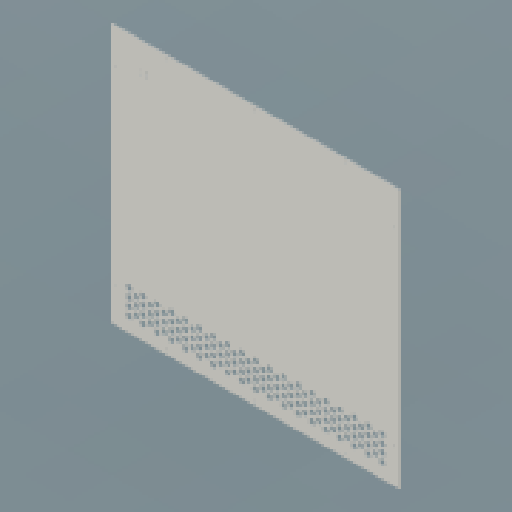
# Autodesk Inventor part: Rear Panel
Saved by Autodesk Inventor 2023.2 (Build 272271000, 271)
## iProperties
Created: 2023-02-06
Part Number: Rear Panel
Material: Aluminum 6061
Document SubType Name: Modeling
Designer: remop
Density: 2.7 g/cm^3
Appearance: Aluminum - Flat
Author: remop
Autodesk Inventor part; units mm, degrees
(part 1 of 2)
ref_plane "YZ Plane" through (0, 0, 0) normal (1, 0, 0) x (0, 1, 0)
ref_plane "XZ Plane" through (0, 0, 0) normal (0, 1, 0) x (-1, 0, 0)
ref_plane "XY Plane" through (0, 0, 0) normal (0, 0, 1) x (1, 0, 0)
sketch "Sketch1" plane through (0, 0, 0) normal (0, 0, 1) x (1, 0, 0)
  line L0 (287.336, -253.0124) -> (287.336, 226.9876) projected
  line L1 (287.336, 226.9876) -> (289.336, 226.9876) projected
  line L2 (289.336, -253.0124) -> (289.336, 226.9876) projected
  line L3 (287.336, -253.0124) -> (289.336, -253.0124) projected
  line L4 (-242.664, 226.9876) -> (-242.664, -253.0124) projected
  line L5 (-242.664, -253.0124) -> (-244.664, -253.0124) projected
  line L6 (-244.664, 226.9876) -> (-244.664, -253.0124) projected
  line L7 (-242.664, 226.9876) -> (-244.664, 226.9876) projected
  line L8 (287.336, 226.9876) -> (-242.664, 226.9876)
  line L9 (-242.664, -253.0124) -> (287.336, -253.0124)
  circle A0 centre (187.336, 219.4876) radius 1.75
  circle A1 centre (-142.664, 219.4876) radius 1.75
  circle A2 centre (22.336, 219.4876) radius 1.75
  circle A3 centre (187.336, -245.5124) radius 1.75
  circle A4 centre (22.336, -245.5124) radius 1.75
  circle A5 centre (-142.664, -245.5124) radius 1.75
  circle A6 centre (279.836, 161.9876) radius 1.75
  circle A7 centre (279.836, -188.0124) radius 1.75
  circle A8 centre (-235.164, -188.0124) radius 1.75
  circle A9 centre (-235.164, 161.9876) radius 1.75
  point P0 (0, 0)
  point P1 (22.336, 226.9876)
  dimension "d0" = 7.5
  dimension "d1" = 100
  dimension "d2" = 100
  dimension "d3" = 3.5
  dimension "d4" = 7.5
  dimension "d7" = 65
  dimension "d8" = 65
  dimension "d10" = 7.5
  dimension "d11" = 7.5
  constraints: 10 centre point, 9 equal radius, 6 horizontal alignment, 6 vertical alignment, 4 end point, 1 horizontal, 1 midpoint, 1 parallel
  measures "d0" distance from line of A0.centre L8
  measures "d1" distance from line of L0 A0.centre
  measures "d2" distance from line of L4 A1.centre
  measures "d3" diameter of A2
  measures "d4" distance from line of L9 A3.centre
  measures "d7" distance from line of A7.centre L9
  measures "d8" distance from line of L8 A6.centre
  measures "d10" distance from line of L4 A9.centre
  measures "d11" distance from line of L0 A6.centre
extrude "Extrusion1" add sketch "Sketch1" against normal blind 2
sketch "Sketch2" plane through (0, 0, 0) normal (0, 0, 1) x (1, 0, 0)
  line L0 (-204.6641, 162.9876) -> (-216.6641, 162.9876) projected
  line L1 (-204.6641, 162.9876) -> (-204.6641, 184.9876) projected
  line L2 (-216.6641, 184.9876) -> (-204.6641, 184.9876) projected
  line L3 (-216.6641, 162.9876) -> (-216.6641, 184.9876) projected
  line L4 (70.3359, 162.9876) -> (-204.6641, 162.9876) projected
  line L5 (70.3359, 162.9876) -> (70.3359, 184.9876) projected
  line L6 (-204.6641, 184.9876) -> (70.3359, 184.9876) projected
  line L7 (-204.6641, 162.9876) -> (-204.6641, 184.9876) projected
  point P0 (0, 0)
  point P1 (-209.6641, 177.4876)
  point P2 (-209.6641, 170.4876)
  point P3 (-199.6641, 170.4876)
  point P4 (-199.6641, 177.4876)
  dimension "d12" = 7
  dimension "d13" = 10
  dimension "d14" = 7.5
  dimension "d15" = 7
  constraints: 2 horizontal alignment, 2 vertical alignment
  measures "d12" distance of point (-199.664, 170.488) point (-199.664, 177.488)
  measures "d13" distance of point (-199.664, 177.488) point (-209.664, 177.488)
  measures "d14" distance from line of L2 point (-209.664, 177.488)
  measures "d15" distance from line of L3 point (-209.664, 177.488)
hole "Hole1" at (-209.6641, 177.4876, 0) at (-209.6641, 170.4876, 0) at (-199.6641, 170.4876, 0) at (-199.6641, 177.4876, 0) direction (0, 0, -1) diameter 3.5 end through all
sketch "Sketch4" plane through (0, 0, -2) normal (0, 0, -1) x (-1, 0, 0)
  circle A0 centre (199.6641, 170.4876) radius 1.75 projected
  circle A1 centre (209.6641, 177.4876) radius 1.75 projected
  circle A2 centre (209.6641, 170.4876) radius 1.75 projected
  circle A3 centre (199.6641, 177.4876) radius 1.75 projected
  line L0 (244.664, 226.9876) -> (-289.336, 226.9876) projected
  line L1 (-289.336, 226.9876) -> (-289.336, -253.0124) projected
  line L2 (-289.336, -253.0124) -> (244.664, -253.0124) projected
  line L3 (244.664, -253.0124) -> (244.664, 226.9876) projected
  circle A4 centre (235.164, 161.9876) radius 1.75 projected
  circle A5 centre (-279.836, -188.0124) radius 1.75 projected
  circle A6 centre (-279.836, 161.9876) radius 1.75 projected
  circle A7 centre (142.664, -245.5124) radius 1.75 projected
  circle A8 centre (-22.336, -245.5124) radius 1.75 projected
  circle A9 centre (-187.336, -245.5124) radius 1.75 projected
  circle A10 centre (-22.336, 219.4876) radius 1.75 projected
  circle A11 centre (142.664, 219.4876) radius 1.75 projected
  circle A12 centre (-187.336, 219.4876) radius 1.75 projected
  circle A13 centre (235.164, -188.0124) radius 1.75 projected
  line L4 (-250.5625, -226.0124) -> (-253.4493, -231.0124)
  line L5 (-253.4493, -231.0124) -> (-259.2228, -231.0124)
  line L6 (-259.2228, -231.0124) -> (-262.1095, -226.0124)
  line L7 (-262.1095, -226.0124) -> (-259.2228, -221.0124)
  line L8 (-259.2228, -221.0124) -> (-253.4493, -221.0124)
  line L9 (-253.4493, -221.0124) -> (-250.5625, -226.0124)
  line L10 (-246.2324, -223.5124) -> (-249.1191, -218.5124)
  line L11 (-249.1191, -218.5124) -> (-246.2324, -213.5124)
  line L12 (-246.2324, -213.5124) -> (-240.4589, -213.5124)
  line L13 (-240.4589, -213.5124) -> (-237.5721, -218.5124)
  line L14 (-237.5721, -218.5124) -> (-240.4589, -223.5124)
  line L15 (-240.4589, -223.5124) -> (-246.2324, -223.5124)
  line L16 (-253.4493, -216.0124) -> (-259.2228, -216.0124)
  line L17 (-259.2228, -216.0124) -> (-262.1095, -211.0124)
  line L18 (-262.1095, -211.0124) -> (-259.2228, -206.0124)
  line L19 (-259.2228, -206.0124) -> (-253.4493, -206.0124)
  line L20 (-253.4493, -206.0124) -> (-250.5625, -211.0124)
  line L21 (-250.5625, -211.0124) -> (-253.4493, -216.0124)
  line L22 (-246.2324, -198.5124) -> (-240.4589, -198.5124)
  line L23 (-249.1191, -203.5124) -> (-246.2324, -198.5124)
  line L24 (-240.4589, -198.5124) -> (-237.5721, -203.5124)
  line L25 (-250.5625, -196.0124) -> (-253.4493, -201.0124)
  line L26 (-253.4493, -191.0124) -> (-250.5625, -196.0124)
  line L27 (-253.4493, -201.0124) -> (-259.2228, -201.0124)
  line L28 (-259.2228, -191.0124) -> (-253.4493, -191.0124)
  line L29 (-262.1095, -196.0124) -> (-259.2228, -191.0124)
  line L30 (-259.2228, -201.0124) -> (-262.1095, -196.0124)
  line L31 (-237.5721, -203.5124) -> (-240.4589, -208.5124)
  line L32 (-240.4589, -208.5124) -> (-246.2324, -208.5124)
  line L33 (-246.2324, -208.5124) -> (-249.1191, -203.5124)
  line L34 (-246.2324, -183.5124) -> (-240.4589, -183.5124)
  line L35 (-249.1191, -188.5124) -> (-246.2324, -183.5124)
  line L36 (-240.4589, -183.5124) -> (-237.5721, -188.5124)
  line L37 (-250.5625, -181.0124) -> (-253.4493, -186.0124)
  line L38 (-253.4493, -176.0124) -> (-250.5625, -181.0124)
  line L39 (-253.4493, -186.0124) -> (-259.2228, -186.0124)
  line L40 (-259.2228, -176.0124) -> (-253.4493, -176.0124)
  line L41 (-262.1095, -181.0124) -> (-259.2228, -176.0124)
  line L42 (-259.2228, -186.0124) -> (-262.1095, -181.0124)
  line L43 (-237.5721, -188.5124) -> (-240.4589, -193.5124)
  line L44 (-240.4589, -193.5124) -> (-246.2324, -193.5124)
  line L45 (-246.2324, -193.5124) -> (-249.1191, -188.5124)
  line L46 (-227.4493, -176.0124) -> (-224.5625, -181.0124)
  line L47 (-233.2228, -176.0124) -> (-227.4493, -176.0124)
  line L48 (-236.1095, -181.0124) -> (-233.2228, -176.0124)
  line L49 (-214.4589, -208.5124) -> (-220.2324, -208.5124)
  line L50 (-220.2324, -198.5124) -> (-214.4589, -198.5124)
  line L51 (-211.5721, -188.5124) -> (-214.4589, -193.5124)
  line L52 (-214.4589, -193.5124) -> (-220.2324, -193.5124)
  line L53 (-214.4589, -183.5124) -> (-211.5721, -188.5124)
  line L54 (-220.2324, -183.5124) -> (-214.4589, -183.5124)
  line L55 (-220.2324, -208.5124) -> (-223.1191, -203.5124)
  line L56 (-223.1191, -203.5124) -> (-220.2324, -198.5124)
  line L57 (-220.2324, -193.5124) -> (-223.1191, -188.5124)
  line L58 (-223.1191, -188.5124) -> (-220.2324, -183.5124)
  line L59 (-224.5625, -211.0124) -> (-227.4493, -216.0124)
  line L60 (-227.4493, -221.0124) -> (-224.5625, -226.0124)
  line L61 (-224.5625, -226.0124) -> (-227.4493, -231.0124)
  line L62 (-233.2228, -221.0124) -> (-227.4493, -221.0124)
  line L63 (-227.4493, -231.0124) -> (-233.2228, -231.0124)
  line L64 (-233.2228, -231.0124) -> (-236.1095, -226.0124)
  line L65 (-236.1095, -226.0124) -> (-233.2228, -221.0124)
  line L66 (-227.4493, -206.0124) -> (-224.5625, -211.0124)
  line L67 (-227.4493, -216.0124) -> (-233.2228, -216.0124)
  line L68 (-233.2228, -216.0124) -> (-236.1095, -211.0124)
  line L69 (-233.2228, -206.0124) -> (-227.4493, -206.0124)
  line L70 (-236.1095, -211.0124) -> (-233.2228, -206.0124)
  line L71 (-223.1191, -218.5124) -> (-220.2324, -213.5124)
  line L72 (-220.2324, -213.5124) -> (-214.4589, -213.5124)
  line L73 (-214.4589, -213.5124) -> (-211.5721, -218.5124)
  line L74 (-214.4589, -223.5124) -> (-220.2324, -223.5124)
  line L75 (-211.5721, -218.5124) -> (-214.4589, -223.5124)
  line L76 (-220.2324, -223.5124) -> (-223.1191, -218.5124)
  line L77 (-224.5625, -181.0124) -> (-227.4493, -186.0124)
  line L78 (-233.2228, -186.0124) -> (-236.1095, -181.0124)
  line L79 (-227.4493, -186.0124) -> (-233.2228, -186.0124)
  line L80 (-227.4493, -191.0124) -> (-224.5625, -196.0124)
  line L81 (-236.1095, -196.0124) -> (-233.2228, -191.0124)
  line L82 (-224.5625, -196.0124) -> (-227.4493, -201.0124)
  line L83 (-233.2228, -201.0124) -> (-236.1095, -196.0124)
  line L84 (-227.4493, -201.0124) -> (-233.2228, -201.0124)
  line L85 (-233.2228, -191.0124) -> (-227.4493, -191.0124)
  line L86 (-211.5721, -203.5124) -> (-214.4589, -208.5124)
  line L87 (-214.4589, -198.5124) -> (-211.5721, -203.5124)
  line L88 (-201.4493, -176.0124) -> (-198.5625, -181.0124)
  line L89 (-207.2228, -176.0124) -> (-201.4493, -176.0124)
  line L90 (-210.1095, -181.0124) -> (-207.2228, -176.0124)
  line L91 (-188.4589, -208.5124) -> (-194.2324, -208.5124)
  line L92 (-194.2324, -198.5124) -> (-188.4589, -198.5124)
  line L93 (-185.5721, -188.5124) -> (-188.4589, -193.5124)
  line L94 (-188.4589, -193.5124) -> (-194.2324, -193.5124)
  line L95 (-188.4589, -183.5124) -> (-185.5721, -188.5124)
  line L96 (-194.2324, -183.5124) -> (-188.4589, -183.5124)
  line L97 (-194.2324, -208.5124) -> (-197.1191, -203.5124)
  line L98 (-197.1191, -203.5124) -> (-194.2324, -198.5124)
  line L99 (-194.2324, -193.5124) -> (-197.1191, -188.5124)
  line L100 (-197.1191, -188.5124) -> (-194.2324, -183.5124)
  line L101 (-198.5625, -211.0124) -> (-201.4493, -216.0124)
  line L102 (-201.4493, -221.0124) -> (-198.5625, -226.0124)
  line L103 (-198.5625, -226.0124) -> (-201.4493, -231.0124)
  line L104 (-207.2228, -221.0124) -> (-201.4493, -221.0124)
  line L105 (-201.4493, -231.0124) -> (-207.2228, -231.0124)
  line L106 (-207.2228, -231.0124) -> (-210.1095, -226.0124)
  line L107 (-210.1095, -226.0124) -> (-207.2228, -221.0124)
  line L108 (-201.4493, -206.0124) -> (-198.5625, -211.0124)
  line L109 (-201.4493, -216.0124) -> (-207.2228, -216.0124)
  line L110 (-207.2228, -216.0124) -> (-210.1095, -211.0124)
  line L111 (-207.2228, -206.0124) -> (-201.4493, -206.0124)
  line L112 (-210.1095, -211.0124) -> (-207.2228, -206.0124)
  line L113 (-197.1191, -218.5124) -> (-194.2324, -213.5124)
  line L114 (-194.2324, -213.5124) -> (-188.4589, -213.5124)
  line L115 (-188.4589, -213.5124) -> (-185.5721, -218.5124)
  line L116 (-188.4589, -223.5124) -> (-194.2324, -223.5124)
  line L117 (-185.5721, -218.5124) -> (-188.4589, -223.5124)
  line L118 (-194.2324, -223.5124) -> (-197.1191, -218.5124)
  line L119 (-198.5625, -181.0124) -> (-201.4493, -186.0124)
  line L120 (-207.2228, -186.0124) -> (-210.1095, -181.0124)
  line L121 (-201.4493, -186.0124) -> (-207.2228, -186.0124)
  line L122 (-201.4493, -191.0124) -> (-198.5625, -196.0124)
  line L123 (-210.1095, -196.0124) -> (-207.2228, -191.0124)
  line L124 (-198.5625, -196.0124) -> (-201.4493, -201.0124)
  line L125 (-207.2228, -201.0124) -> (-210.1095, -196.0124)
  line L126 (-201.4493, -201.0124) -> (-207.2228, -201.0124)
  line L127 (-207.2228, -191.0124) -> (-201.4493, -191.0124)
  line L128 (-185.5721, -203.5124) -> (-188.4589, -208.5124)
  line L129 (-188.4589, -198.5124) -> (-185.5721, -203.5124)
  line L130 (-175.4493, -176.0124) -> (-172.5625, -181.0124)
  line L131 (-181.2228, -176.0124) -> (-175.4493, -176.0124)
  line L132 (-184.1095, -181.0124) -> (-181.2228, -176.0124)
  line L133 (-162.4589, -208.5124) -> (-168.2324, -208.5124)
  line L134 (-168.2324, -198.5124) -> (-162.4589, -198.5124)
  line L135 (-159.5721, -188.5124) -> (-162.4589, -193.5124)
  line L136 (-162.4589, -193.5124) -> (-168.2324, -193.5124)
  line L137 (-162.4589, -183.5124) -> (-159.5721, -188.5124)
  line L138 (-168.2324, -183.5124) -> (-162.4589, -183.5124)
  line L139 (-168.2324, -208.5124) -> (-171.1191, -203.5124)
  line L140 (-171.1191, -203.5124) -> (-168.2324, -198.5124)
  line L141 (-168.2324, -193.5124) -> (-171.1191, -188.5124)
  line L142 (-171.1191, -188.5124) -> (-168.2324, -183.5124)
  line L143 (-172.5625, -211.0124) -> (-175.4493, -216.0124)
  line L144 (-175.4493, -221.0124) -> (-172.5625, -226.0124)
  line L145 (-172.5625, -226.0124) -> (-175.4493, -231.0124)
  line L146 (-181.2228, -221.0124) -> (-175.4493, -221.0124)
  line L147 (-175.4493, -231.0124) -> (-181.2228, -231.0124)
  line L148 (-181.2228, -231.0124) -> (-184.1095, -226.0124)
  line L149 (-184.1095, -226.0124) -> (-181.2228, -221.0124)
  line L150 (-175.4493, -206.0124) -> (-172.5625, -211.0124)
  line L151 (-175.4493, -216.0124) -> (-181.2228, -216.0124)
  line L152 (-181.2228, -216.0124) -> (-184.1095, -211.0124)
  line L153 (-181.2228, -206.0124) -> (-175.4493, -206.0124)
  line L154 (-184.1095, -211.0124) -> (-181.2228, -206.0124)
  line L155 (-171.1191, -218.5124) -> (-168.2324, -213.5124)
  line L156 (-168.2324, -213.5124) -> (-162.4589, -213.5124)
  line L157 (-162.4589, -213.5124) -> (-159.5721, -218.5124)
  line L158 (-162.4589, -223.5124) -> (-168.2324, -223.5124)
  line L159 (-159.5721, -218.5124) -> (-162.4589, -223.5124)
  line L160 (-168.2324, -223.5124) -> (-171.1191, -218.5124)
  line L161 (-172.5625, -181.0124) -> (-175.4493, -186.0124)
  line L162 (-181.2228, -186.0124) -> (-184.1095, -181.0124)
  line L163 (-175.4493, -186.0124) -> (-181.2228, -186.0124)
  line L164 (-175.4493, -191.0124) -> (-172.5625, -196.0124)
  line L165 (-184.1095, -196.0124) -> (-181.2228, -191.0124)
  line L166 (-172.5625, -196.0124) -> (-175.4493, -201.0124)
  line L167 (-181.2228, -201.0124) -> (-184.1095, -196.0124)
  line L168 (-175.4493, -201.0124) -> (-181.2228, -201.0124)
  line L169 (-181.2228, -191.0124) -> (-175.4493, -191.0124)
  line L170 (-159.5721, -203.5124) -> (-162.4589, -208.5124)
  line L171 (-162.4589, -198.5124) -> (-159.5721, -203.5124)
  line L172 (-149.4493, -176.0124) -> (-146.5625, -181.0124)
  line L173 (-155.2228, -176.0124) -> (-149.4493, -176.0124)
  line L174 (-158.1095, -181.0124) -> (-155.2228, -176.0124)
  line L175 (-136.4589, -208.5124) -> (-142.2324, -208.5124)
  line L176 (-142.2324, -198.5124) -> (-136.4589, -198.5124)
  line L177 (-133.5721, -188.5124) -> (-136.4589, -193.5124)
  line L178 (-136.4589, -193.5124) -> (-142.2324, -193.5124)
  line L179 (-136.4589, -183.5124) -> (-133.5721, -188.5124)
  line L180 (-142.2324, -183.5124) -> (-136.4589, -183.5124)
  line L181 (-142.2324, -208.5124) -> (-145.1191, -203.5124)
  line L182 (-145.1191, -203.5124) -> (-142.2324, -198.5124)
  line L183 (-142.2324, -193.5124) -> (-145.1191, -188.5124)
  line L184 (-145.1191, -188.5124) -> (-142.2324, -183.5124)
  line L185 (-146.5625, -211.0124) -> (-149.4493, -216.0124)
  line L186 (-149.4493, -221.0124) -> (-146.5625, -226.0124)
  line L187 (-146.5625, -226.0124) -> (-149.4493, -231.0124)
  line L188 (-155.2228, -221.0124) -> (-149.4493, -221.0124)
  line L189 (-149.4493, -231.0124) -> (-155.2228, -231.0124)
  line L190 (-155.2228, -231.0124) -> (-158.1095, -226.0124)
  line L191 (-158.1095, -226.0124) -> (-155.2228, -221.0124)
  line L192 (-149.4493, -206.0124) -> (-146.5625, -211.0124)
  line L193 (-149.4493, -216.0124) -> (-155.2228, -216.0124)
  line L194 (-155.2228, -216.0124) -> (-158.1095, -211.0124)
  line L195 (-155.2228, -206.0124) -> (-149.4493, -206.0124)
  line L196 (-158.1095, -211.0124) -> (-155.2228, -206.0124)
  line L197 (-145.1191, -218.5124) -> (-142.2324, -213.5124)
  line L198 (-142.2324, -213.5124) -> (-136.4589, -213.5124)
  line L199 (-136.4589, -213.5124) -> (-133.5721, -218.5124)
  line L200 (-136.4589, -223.5124) -> (-142.2324, -223.5124)
  line L201 (-133.5721, -218.5124) -> (-136.4589, -223.5124)
  line L202 (-142.2324, -223.5124) -> (-145.1191, -218.5124)
  line L203 (-146.5625, -181.0124) -> (-149.4493, -186.0124)
  line L204 (-155.2228, -186.0124) -> (-158.1095, -181.0124)
  line L205 (-149.4493, -186.0124) -> (-155.2228, -186.0124)
  line L206 (-149.4493, -191.0124) -> (-146.5625, -196.0124)
  line L207 (-158.1095, -196.0124) -> (-155.2228, -191.0124)
  line L208 (-146.5625, -196.0124) -> (-149.4493, -201.0124)
  line L209 (-155.2228, -201.0124) -> (-158.1095, -196.0124)
  line L210 (-149.4493, -201.0124) -> (-155.2228, -201.0124)
  line L211 (-155.2228, -191.0124) -> (-149.4493, -191.0124)
  line L212 (-133.5721, -203.5124) -> (-136.4589, -208.5124)
  line L213 (-136.4589, -198.5124) -> (-133.5721, -203.5124)
  line L214 (-123.4493, -176.0124) -> (-120.5625, -181.0124)
  line L215 (-129.2228, -176.0124) -> (-123.4493, -176.0124)
  line L216 (-132.1095, -181.0124) -> (-129.2228, -176.0124)
  line L217 (-110.4589, -208.5124) -> (-116.2324, -208.5124)
  line L218 (-116.2324, -198.5124) -> (-110.4589, -198.5124)
  line L219 (-107.5721, -188.5124) -> (-110.4589, -193.5124)
  line L220 (-110.4589, -193.5124) -> (-116.2324, -193.5124)
  line L221 (-110.4589, -183.5124) -> (-107.5721, -188.5124)
  line L222 (-116.2324, -183.5124) -> (-110.4589, -183.5124)
  line L223 (-116.2324, -208.5124) -> (-119.1191, -203.5124)
  line L224 (-119.1191, -203.5124) -> (-116.2324, -198.5124)
  line L225 (-116.2324, -193.5124) -> (-119.1191, -188.5124)
  line L226 (-119.1191, -188.5124) -> (-116.2324, -183.5124)
  line L227 (-120.5625, -211.0124) -> (-123.4493, -216.0124)
  line L228 (-123.4493, -221.0124) -> (-120.5625, -226.0124)
  line L229 (-120.5625, -226.0124) -> (-123.4493, -231.0124)
  line L230 (-129.2228, -221.0124) -> (-123.4493, -221.0124)
  line L231 (-123.4493, -231.0124) -> (-129.2228, -231.0124)
  line L232 (-129.2228, -231.0124) -> (-132.1095, -226.0124)
  line L233 (-132.1095, -226.0124) -> (-129.2228, -221.0124)
  line L234 (-123.4493, -206.0124) -> (-120.5625, -211.0124)
  line L235 (-123.4493, -216.0124) -> (-129.2228, -216.0124)
  line L236 (-129.2228, -216.0124) -> (-132.1095, -211.0124)
  line L237 (-129.2228, -206.0124) -> (-123.4493, -206.0124)
  line L238 (-132.1095, -211.0124) -> (-129.2228, -206.0124)
  line L239 (-119.1191, -218.5124) -> (-116.2324, -213.5124)
  line L240 (-116.2324, -213.5124) -> (-110.4589, -213.5124)
  line L241 (-110.4589, -213.5124) -> (-107.5721, -218.5124)
  line L242 (-110.4589, -223.5124) -> (-116.2324, -223.5124)
  line L243 (-107.5721, -218.5124) -> (-110.4589, -223.5124)
  line L244 (-116.2324, -223.5124) -> (-119.1191, -218.5124)
  line L245 (-120.5625, -181.0124) -> (-123.4493, -186.0124)
  line L246 (-129.2228, -186.0124) -> (-132.1095, -181.0124)
  line L247 (-123.4493, -186.0124) -> (-129.2228, -186.0124)
  line L248 (-123.4493, -191.0124) -> (-120.5625, -196.0124)
  line L249 (-132.1095, -196.0124) -> (-129.2228, -191.0124)
  line L250 (-120.5625, -196.0124) -> (-123.4493, -201.0124)
  line L251 (-129.2228, -201.0124) -> (-132.1095, -196.0124)
  line L252 (-123.4493, -201.0124) -> (-129.2228, -201.0124)
  line L253 (-129.2228, -191.0124) -> (-123.4493, -191.0124)
  line L254 (-107.5721, -203.5124) -> (-110.4589, -208.5124)
  line L255 (-110.4589, -198.5124) -> (-107.5721, -203.5124)
  line L256 (-97.4493, -176.0124) -> (-94.5625, -181.0124)
  line L257 (-103.2228, -176.0124) -> (-97.4493, -176.0124)
  line L258 (-106.1095, -181.0124) -> (-103.2228, -176.0124)
  line L259 (-84.4589, -208.5124) -> (-90.2324, -208.5124)
  line L260 (-90.2324, -198.5124) -> (-84.4589, -198.5124)
  line L261 (-81.5721, -188.5124) -> (-84.4589, -193.5124)
  line L262 (-84.4589, -193.5124) -> (-90.2324, -193.5124)
  line L263 (-84.4589, -183.5124) -> (-81.5721, -188.5124)
  line L264 (-90.2324, -183.5124) -> (-84.4589, -183.5124)
  line L265 (-90.2324, -208.5124) -> (-93.1191, -203.5124)
  line L266 (-93.1191, -203.5124) -> (-90.2324, -198.5124)
  line L267 (-90.2324, -193.5124) -> (-93.1191, -188.5124)
  line L268 (-93.1191, -188.5124) -> (-90.2324, -183.5124)
  line L269 (-94.5625, -211.0124) -> (-97.4493, -216.0124)
  line L270 (-97.4493, -221.0124) -> (-94.5625, -226.0124)
  line L271 (-94.5625, -226.0124) -> (-97.4493, -231.0124)
  line L272 (-103.2228, -221.0124) -> (-97.4493, -221.0124)
  line L273 (-97.4493, -231.0124) -> (-103.2228, -231.0124)
  line L274 (-103.2228, -231.0124) -> (-106.1095, -226.0124)
  line L275 (-106.1095, -226.0124) -> (-103.2228, -221.0124)
  line L276 (-97.4493, -206.0124) -> (-94.5625, -211.0124)
  line L277 (-97.4493, -216.0124) -> (-103.2228, -216.0124)
  line L278 (-103.2228, -216.0124) -> (-106.1095, -211.0124)
  line L279 (-103.2228, -206.0124) -> (-97.4493, -206.0124)
  line L280 (-106.1095, -211.0124) -> (-103.2228, -206.0124)
  line L281 (-93.1191, -218.5124) -> (-90.2324, -213.5124)
  line L282 (-90.2324, -213.5124) -> (-84.4589, -213.5124)
  line L283 (-84.4589, -213.5124) -> (-81.5721, -218.5124)
  line L284 (-84.4589, -223.5124) -> (-90.2324, -223.5124)
  line L285 (-81.5721, -218.5124) -> (-84.4589, -223.5124)
  line L286 (-90.2324, -223.5124) -> (-93.1191, -218.5124)
  line L287 (-94.5625, -181.0124) -> (-97.4493, -186.0124)
  line L288 (-103.2228, -186.0124) -> (-106.1095, -181.0124)
  line L289 (-97.4493, -186.0124) -> (-103.2228, -186.0124)
  line L290 (-97.4493, -191.0124) -> (-94.5625, -196.0124)
  line L291 (-106.1095, -196.0124) -> (-103.2228, -191.0124)
  line L292 (-94.5625, -196.0124) -> (-97.4493, -201.0124)
  line L293 (-103.2228, -201.0124) -> (-106.1095, -196.0124)
  line L294 (-97.4493, -201.0124) -> (-103.2228, -201.0124)
  line L295 (-103.2228, -191.0124) -> (-97.4493, -191.0124)
  line L296 (-81.5721, -203.5124) -> (-84.4589, -208.5124)
  line L297 (-84.4589, -198.5124) -> (-81.5721, -203.5124)
  line L298 (-71.4493, -176.0124) -> (-68.5625, -181.0124)
  line L299 (-77.2228, -176.0124) -> (-71.4493, -176.0124)
  line L300 (-80.1095, -181.0124) -> (-77.2228, -176.0124)
  line L301 (-58.4589, -208.5124) -> (-64.2324, -208.5124)
  line L302 (-64.2324, -198.5124) -> (-58.4589, -198.5124)
  line L303 (-55.5721, -188.5124) -> (-58.4589, -193.5124)
  line L304 (-58.4589, -193.5124) -> (-64.2324, -193.5124)
  line L305 (-58.4589, -183.5124) -> (-55.5721, -188.5124)
  line L306 (-64.2324, -183.5124) -> (-58.4589, -183.5124)
  line L307 (-64.2324, -208.5124) -> (-67.1191, -203.5124)
  line L308 (-67.1191, -203.5124) -> (-64.2324, -198.5124)
  line L309 (-64.2324, -193.5124) -> (-67.1191, -188.5124)
  line L310 (-67.1191, -188.5124) -> (-64.2324, -183.5124)
  line L311 (-68.5625, -211.0124) -> (-71.4493, -216.0124)
  line L312 (-71.4493, -221.0124) -> (-68.5625, -226.0124)
  line L313 (-68.5625, -226.0124) -> (-71.4493, -231.0124)
  line L314 (-77.2228, -221.0124) -> (-71.4493, -221.0124)
  line L315 (-71.4493, -231.0124) -> (-77.2228, -231.0124)
  line L316 (-77.2228, -231.0124) -> (-80.1095, -226.0124)
  line L317 (-80.1095, -226.0124) -> (-77.2228, -221.0124)
  line L318 (-71.4493, -206.0124) -> (-68.5625, -211.0124)
  line L319 (-71.4493, -216.0124) -> (-77.2228, -216.0124)
  line L320 (-77.2228, -216.0124) -> (-80.1095, -211.0124)
  line L321 (-77.2228, -206.0124) -> (-71.4493, -206.0124)
  line L322 (-80.1095, -211.0124) -> (-77.2228, -206.0124)
  line L323 (-67.1191, -218.5124) -> (-64.2324, -213.5124)
  line L324 (-64.2324, -213.5124) -> (-58.4589, -213.5124)
  line L325 (-58.4589, -213.5124) -> (-55.5721, -218.5124)
  line L326 (-58.4589, -223.5124) -> (-64.2324, -223.5124)
  line L327 (-55.5721, -218.5124) -> (-58.4589, -223.5124)
  line L328 (-64.2324, -223.5124) -> (-67.1191, -218.5124)
  line L329 (-68.5625, -181.0124) -> (-71.4493, -186.0124)
  line L330 (-77.2228, -186.0124) -> (-80.1095, -181.0124)
  line L331 (-71.4493, -186.0124) -> (-77.2228, -186.0124)
  line L332 (-71.4493, -191.0124) -> (-68.5625, -196.0124)
  line L333 (-80.1095, -196.0124) -> (-77.2228, -191.0124)
  line L334 (-68.5625, -196.0124) -> (-71.4493, -201.0124)
  line L335 (-77.2228, -201.0124) -> (-80.1095, -196.0124)
  line L336 (-71.4493, -201.0124) -> (-77.2228, -201.0124)
  line L337 (-77.2228, -191.0124) -> (-71.4493, -191.0124)
  line L338 (-55.5721, -203.5124) -> (-58.4589, -208.5124)
  line L339 (-58.4589, -198.5124) -> (-55.5721, -203.5124)
  line L340 (-45.4493, -176.0124) -> (-42.5625, -181.0124)
  line L341 (-51.2228, -176.0124) -> (-45.4493, -176.0124)
  line L342 (-54.1095, -181.0124) -> (-51.2228, -176.0124)
  line L343 (-32.4589, -208.5124) -> (-38.2324, -208.5124)
  line L344 (-38.2324, -198.5124) -> (-32.4589, -198.5124)
  line L345 (-29.5721, -188.5124) -> (-32.4589, -193.5124)
  line L346 (-32.4589, -193.5124) -> (-38.2324, -193.5124)
  line L347 (-32.4589, -183.5124) -> (-29.5721, -188.5124)
  line L348 (-38.2324, -183.5124) -> (-32.4589, -183.5124)
  line L349 (-38.2324, -208.5124) -> (-41.1191, -203.5124)
  line L350 (-41.1191, -203.5124) -> (-38.2324, -198.5124)
  line L351 (-38.2324, -193.5124) -> (-41.1191, -188.5124)
  line L352 (-41.1191, -188.5124) -> (-38.2324, -183.5124)
  line L353 (-42.5625, -211.0124) -> (-45.4493, -216.0124)
  line L354 (-45.4493, -221.0124) -> (-42.5625, -226.0124)
  line L355 (-42.5625, -226.0124) -> (-45.4493, -231.0124)
  line L356 (-51.2228, -221.0124) -> (-45.4493, -221.0124)
  line L357 (-45.4493, -231.0124) -> (-51.2228, -231.0124)
  line L358 (-51.2228, -231.0124) -> (-54.1095, -226.0124)
  line L359 (-54.1095, -226.0124) -> (-51.2228, -221.0124)
  line L360 (-45.4493, -206.0124) -> (-42.5625, -211.0124)
  line L361 (-45.4493, -216.0124) -> (-51.2228, -216.0124)
  line L362 (-51.2228, -216.0124) -> (-54.1095, -211.0124)
  line L363 (-51.2228, -206.0124) -> (-45.4493, -206.0124)
  line L364 (-54.1095, -211.0124) -> (-51.2228, -206.0124)
  line L365 (-41.1191, -218.5124) -> (-38.2324, -213.5124)
  line L366 (-38.2324, -213.5124) -> (-32.4589, -213.5124)
  line L367 (-32.4589, -213.5124) -> (-29.5721, -218.5124)
  line L368 (-32.4589, -223.5124) -> (-38.2324, -223.5124)
  line L369 (-29.5721, -218.5124) -> (-32.4589, -223.5124)
  line L370 (-38.2324, -223.5124) -> (-41.1191, -218.5124)
  line L371 (-42.5625, -181.0124) -> (-45.4493, -186.0124)
  line L372 (-51.2228, -186.0124) -> (-54.1095, -181.0124)
  line L373 (-45.4493, -186.0124) -> (-51.2228, -186.0124)
  line L374 (-45.4493, -191.0124) -> (-42.5625, -196.0124)
  line L375 (-54.1095, -196.0124) -> (-51.2228, -191.0124)
  line L376 (-42.5625, -196.0124) -> (-45.4493, -201.0124)
  line L377 (-51.2228, -201.0124) -> (-54.1095, -196.0124)
  line L378 (-45.4493, -201.0124) -> (-51.2228, -201.0124)
  line L379 (-51.2228, -191.0124) -> (-45.4493, -191.0124)
  line L380 (-29.5721, -203.5124) -> (-32.4589, -208.5124)
  line L381 (-32.4589, -198.5124) -> (-29.5721, -203.5124)
  line L382 (-19.4493, -176.0124) -> (-16.5625, -181.0124)
  line L383 (-25.2228, -176.0124) -> (-19.4493, -176.0124)
  line L384 (-28.1095, -181.0124) -> (-25.2228, -176.0124)
  line L385 (-6.4589, -208.5124) -> (-12.2324, -208.5124)
  line L386 (-12.2324, -198.5124) -> (-6.4589, -198.5124)
  line L387 (-3.5721, -188.5124) -> (-6.4589, -193.5124)
  line L388 (-6.4589, -193.5124) -> (-12.2324, -193.5124)
  line L389 (-6.4589, -183.5124) -> (-3.5721, -188.5124)
  line L390 (-12.2324, -183.5124) -> (-6.4589, -183.5124)
  line L391 (-12.2324, -208.5124) -> (-15.1191, -203.5124)
  line L392 (-15.1191, -203.5124) -> (-12.2324, -198.5124)
  line L393 (-12.2324, -193.5124) -> (-15.1191, -188.5124)
  line L394 (-15.1191, -188.5124) -> (-12.2324, -183.5124)
  line L395 (-16.5625, -211.0124) -> (-19.4493, -216.0124)
  line L396 (-19.4493, -221.0124) -> (-16.5625, -226.0124)
  line L397 (-16.5625, -226.0124) -> (-19.4493, -231.0124)
  line L398 (-25.2228, -221.0124) -> (-19.4493, -221.0124)
  line L399 (-19.4493, -231.0124) -> (-25.2228, -231.0124)
  line L400 (-25.2228, -231.0124) -> (-28.1095, -226.0124)
  line L401 (-28.1095, -226.0124) -> (-25.2228, -221.0124)
  line L402 (-19.4493, -206.0124) -> (-16.5625, -211.0124)
  line L403 (-19.4493, -216.0124) -> (-25.2228, -216.0124)
  line L404 (-25.2228, -216.0124) -> (-28.1095, -211.0124)
  line L405 (-25.2228, -206.0124) -> (-19.4493, -206.0124)
  line L406 (-28.1095, -211.0124) -> (-25.2228, -206.0124)
  line L407 (-15.1191, -218.5124) -> (-12.2324, -213.5124)
  line L408 (-12.2324, -213.5124) -> (-6.4589, -213.5124)
  line L409 (-6.4589, -213.5124) -> (-3.5721, -218.5124)
  line L410 (-6.4589, -223.5124) -> (-12.2324, -223.5124)
  line L411 (-3.5721, -218.5124) -> (-6.4589, -223.5124)
  line L412 (-12.2324, -223.5124) -> (-15.1191, -218.5124)
  line L413 (-16.5625, -181.0124) -> (-19.4493, -186.0124)
  line L414 (-25.2228, -186.0124) -> (-28.1095, -181.0124)
  line L415 (-19.4493, -186.0124) -> (-25.2228, -186.0124)
  line L416 (-19.4493, -191.0124) -> (-16.5625, -196.0124)
  line L417 (-28.1095, -196.0124) -> (-25.2228, -191.0124)
  line L418 (-16.5625, -196.0124) -> (-19.4493, -201.0124)
  line L419 (-25.2228, -201.0124) -> (-28.1095, -196.0124)
  line L420 (-19.4493, -201.0124) -> (-25.2228, -201.0124)
  line L421 (-25.2228, -191.0124) -> (-19.4493, -191.0124)
  line L422 (-3.5721, -203.5124) -> (-6.4589, -208.5124)
  line L423 (-6.4589, -198.5124) -> (-3.5721, -203.5124)
  line L424 (6.5507, -176.0124) -> (9.4375, -181.0124)
  line L425 (0.7772, -176.0124) -> (6.5507, -176.0124)
  line L426 (-2.1095, -181.0124) -> (0.7772, -176.0124)
  line L427 (19.5411, -208.5124) -> (13.7676, -208.5124)
  line L428 (13.7676, -198.5124) -> (19.5411, -198.5124)
  line L429 (22.4279, -188.5124) -> (19.5411, -193.5124)
  line L430 (19.5411, -193.5124) -> (13.7676, -193.5124)
  line L431 (19.5411, -183.5124) -> (22.4279, -188.5124)
  line L432 (13.7676, -183.5124) -> (19.5411, -183.5124)
  line L433 (13.7676, -208.5124) -> (10.8809, -203.5124)
  line L434 (10.8809, -203.5124) -> (13.7676, -198.5124)
  line L435 (13.7676, -193.5124) -> (10.8809, -188.5124)
  line L436 (10.8809, -188.5124) -> (13.7676, -183.5124)
  line L437 (9.4375, -211.0124) -> (6.5507, -216.0124)
  line L438 (6.5507, -221.0124) -> (9.4375, -226.0124)
  line L439 (9.4375, -226.0124) -> (6.5507, -231.0124)
  line L440 (0.7772, -221.0124) -> (6.5507, -221.0124)
  line L441 (6.5507, -231.0124) -> (0.7772, -231.0124)
  line L442 (0.7772, -231.0124) -> (-2.1095, -226.0124)
  line L443 (-2.1095, -226.0124) -> (0.7772, -221.0124)
  line L444 (6.5507, -206.0124) -> (9.4375, -211.0124)
  line L445 (6.5507, -216.0124) -> (0.7772, -216.0124)
  line L446 (0.7772, -216.0124) -> (-2.1095, -211.0124)
  line L447 (0.7772, -206.0124) -> (6.5507, -206.0124)
  line L448 (-2.1095, -211.0124) -> (0.7772, -206.0124)
  line L449 (10.8809, -218.5124) -> (13.7676, -213.5124)
  line L450 (13.7676, -213.5124) -> (19.5411, -213.5124)
  line L451 (19.5411, -213.5124) -> (22.4279, -218.5124)
  line L452 (19.5411, -223.5124) -> (13.7676, -223.5124)
  line L453 (22.4279, -218.5124) -> (19.5411, -223.5124)
  line L454 (13.7676, -223.5124) -> (10.8809, -218.5124)
  line L455 (9.4375, -181.0124) -> (6.5507, -186.0124)
  line L456 (0.7772, -186.0124) -> (-2.1095, -181.0124)
  line L457 (6.5507, -186.0124) -> (0.7772, -186.0124)
  line L458 (6.5507, -191.0124) -> (9.4375, -196.0124)
  line L459 (-2.1095, -196.0124) -> (0.7772, -191.0124)
  line L460 (9.4375, -196.0124) -> (6.5507, -201.0124)
  line L461 (0.7772, -201.0124) -> (-2.1095, -196.0124)
  line L462 (6.5507, -201.0124) -> (0.7772, -201.0124)
  line L463 (0.7772, -191.0124) -> (6.5507, -191.0124)
  line L464 (22.4279, -203.5124) -> (19.5411, -208.5124)
  line L465 (19.5411, -198.5124) -> (22.4279, -203.5124)
  line L466 (32.5507, -176.0124) -> (35.4375, -181.0124)
  line L467 (26.7772, -176.0124) -> (32.5507, -176.0124)
  line L468 (23.8905, -181.0124) -> (26.7772, -176.0124)
  line L469 (45.5411, -208.5124) -> (39.7676, -208.5124)
  line L470 (39.7676, -198.5124) -> (45.5411, -198.5124)
  line L471 (48.4279, -188.5124) -> (45.5411, -193.5124)
  line L472 (45.5411, -193.5124) -> (39.7676, -193.5124)
  line L473 (45.5411, -183.5124) -> (48.4279, -188.5124)
  line L474 (39.7676, -183.5124) -> (45.5411, -183.5124)
  line L475 (39.7676, -208.5124) -> (36.8809, -203.5124)
  line L476 (36.8809, -203.5124) -> (39.7676, -198.5124)
  line L477 (39.7676, -193.5124) -> (36.8809, -188.5124)
  line L478 (36.8809, -188.5124) -> (39.7676, -183.5124)
  line L479 (35.4375, -211.0124) -> (32.5507, -216.0124)
  line L480 (32.5507, -221.0124) -> (35.4375, -226.0124)
  line L481 (35.4375, -226.0124) -> (32.5507, -231.0124)
  line L482 (26.7772, -221.0124) -> (32.5507, -221.0124)
  line L483 (32.5507, -231.0124) -> (26.7772, -231.0124)
  line L484 (26.7772, -231.0124) -> (23.8905, -226.0124)
  line L485 (23.8905, -226.0124) -> (26.7772, -221.0124)
  line L486 (32.5507, -206.0124) -> (35.4375, -211.0124)
  line L487 (32.5507, -216.0124) -> (26.7772, -216.0124)
  line L488 (26.7772, -216.0124) -> (23.8905, -211.0124)
  line L489 (26.7772, -206.0124) -> (32.5507, -206.0124)
  line L490 (23.8905, -211.0124) -> (26.7772, -206.0124)
  line L491 (36.8809, -218.5124) -> (39.7676, -213.5124)
  line L492 (39.7676, -213.5124) -> (45.5411, -213.5124)
  line L493 (45.5411, -213.5124) -> (48.4279, -218.5124)
  line L494 (45.5411, -223.5124) -> (39.7676, -223.5124)
  line L495 (48.4279, -218.5124) -> (45.5411, -223.5124)
  line L496 (39.7676, -223.5124) -> (36.8809, -218.5124)
  line L497 (35.4375, -181.0124) -> (32.5507, -186.0124)
  line L498 (26.7772, -186.0124) -> (23.8905, -181.0124)
  line L499 (32.5507, -186.0124) -> (26.7772, -186.0124)
  line L500 (32.5507, -191.0124) -> (35.4375, -196.0124)
  line L501 (23.8905, -196.0124) -> (26.7772, -191.0124)
  line L502 (35.4375, -196.0124) -> (32.5507, -201.0124)
  line L503 (26.7772, -201.0124) -> (23.8905, -196.0124)
  line L504 (32.5507, -201.0124) -> (26.7772, -201.0124)
  line L505 (26.7772, -191.0124) -> (32.5507, -191.0124)
  line L506 (48.4279, -203.5124) -> (45.5411, -208.5124)
  line L507 (45.5411, -198.5124) -> (48.4279, -203.5124)
  line L508 (58.5507, -176.0124) -> (61.4375, -181.0124)
  line L509 (52.7772, -176.0124) -> (58.5507, -176.0124)
  line L510 (49.8905, -181.0124) -> (52.7772, -176.0124)
  line L511 (71.5411, -208.5124) -> (65.7676, -208.5124)
  line L512 (65.7676, -198.5124) -> (71.5411, -198.5124)
  line L513 (74.4279, -188.5124) -> (71.5411, -193.5124)
  line L514 (71.5411, -193.5124) -> (65.7676, -193.5124)
  line L515 (71.5411, -183.5124) -> (74.4279, -188.5124)
  line L516 (65.7676, -183.5124) -> (71.5411, -183.5124)
  line L517 (65.7676, -208.5124) -> (62.8809, -203.5124)
  line L518 (62.8809, -203.5124) -> (65.7676, -198.5124)
  line L519 (65.7676, -193.5124) -> (62.8809, -188.5124)
  line L520 (62.8809, -188.5124) -> (65.7676, -183.5124)
  line L521 (61.4375, -211.0124) -> (58.5507, -216.0124)
  line L522 (58.5507, -221.0124) -> (61.4375, -226.0124)
  line L523 (61.4375, -226.0124) -> (58.5507, -231.0124)
  line L524 (52.7772, -221.0124) -> (58.5507, -221.0124)
  line L525 (58.5507, -231.0124) -> (52.7772, -231.0124)
  line L526 (52.7772, -231.0124) -> (49.8905, -226.0124)
  line L527 (49.8905, -226.0124) -> (52.7772, -221.0124)
  line L528 (58.5507, -206.0124) -> (61.4375, -211.0124)
  line L529 (58.5507, -216.0124) -> (52.7772, -216.0124)
  line L530 (52.7772, -216.0124) -> (49.8905, -211.0124)
  line L531 (52.7772, -206.0124) -> (58.5507, -206.0124)
  line L532 (49.8905, -211.0124) -> (52.7772, -206.0124)
  line L533 (62.8809, -218.5124) -> (65.7676, -213.5124)
  line L534 (65.7676, -213.5124) -> (71.5411, -213.5124)
  line L535 (71.5411, -213.5124) -> (74.4279, -218.5124)
  line L536 (71.5411, -223.5124) -> (65.7676, -223.5124)
  line L537 (74.4279, -218.5124) -> (71.5411, -223.5124)
  line L538 (65.7676, -223.5124) -> (62.8809, -218.5124)
  line L539 (61.4375, -181.0124) -> (58.5507, -186.0124)
  line L540 (52.7772, -186.0124) -> (49.8905, -181.0124)
  line L541 (58.5507, -186.0124) -> (52.7772, -186.0124)
  line L542 (58.5507, -191.0124) -> (61.4375, -196.0124)
  line L543 (49.8905, -196.0124) -> (52.7772, -191.0124)
  line L544 (61.4375, -196.0124) -> (58.5507, -201.0124)
  line L545 (52.7772, -201.0124) -> (49.8905, -196.0124)
  line L546 (58.5507, -201.0124) -> (52.7772, -201.0124)
  line L547 (52.7772, -191.0124) -> (58.5507, -191.0124)
  line L548 (74.4279, -203.5124) -> (71.5411, -208.5124)
  line L549 (71.5411, -198.5124) -> (74.4279, -203.5124)
  line L550 (84.5507, -176.0124) -> (87.4375, -181.0124)
  line L551 (78.7772, -176.0124) -> (84.5507, -176.0124)
  line L552 (75.8905, -181.0124) -> (78.7772, -176.0124)
  line L553 (97.5411, -208.5124) -> (91.7676, -208.5124)
  line L554 (91.7676, -198.5124) -> (97.5411, -198.5124)
  line L555 (100.4279, -188.5124) -> (97.5411, -193.5124)
  line L556 (97.5411, -193.5124) -> (91.7676, -193.5124)
  line L557 (97.5411, -183.5124) -> (100.4279, -188.5124)
  line L558 (91.7676, -183.5124) -> (97.5411, -183.5124)
  line L559 (91.7676, -208.5124) -> (88.8809, -203.5124)
  line L560 (88.8809, -203.5124) -> (91.7676, -198.5124)
  line L561 (91.7676, -193.5124) -> (88.8809, -188.5124)
  line L562 (88.8809, -188.5124) -> (91.7676, -183.5124)
  line L563 (87.4375, -211.0124) -> (84.5507, -216.0124)
  line L564 (84.5507, -221.0124) -> (87.4375, -226.0124)
  line L565 (87.4375, -226.0124) -> (84.5507, -231.0124)
  line L566 (78.7772, -221.0124) -> (84.5507, -221.0124)
  line L567 (84.5507, -231.0124) -> (78.7772, -231.0124)
  line L568 (78.7772, -231.0124) -> (75.8905, -226.0124)
  line L569 (75.8905, -226.0124) -> (78.7772, -221.0124)
  line L570 (84.5507, -206.0124) -> (87.4375, -211.0124)
  line L571 (84.5507, -216.0124) -> (78.7772, -216.0124)
  line L572 (78.7772, -216.0124) -> (75.8905, -211.0124)
  line L573 (78.7772, -206.0124) -> (84.5507, -206.0124)
  line L574 (75.8905, -211.0124) -> (78.7772, -206.0124)
  line L575 (88.8809, -218.5124) -> (91.7676, -213.5124)
  line L576 (91.7676, -213.5124) -> (97.5411, -213.5124)
  line L577 (97.5411, -213.5124) -> (100.4279, -218.5124)
  line L578 (97.5411, -223.5124) -> (91.7676, -223.5124)
  line L579 (100.4279, -218.5124) -> (97.5411, -223.5124)
  line L580 (91.7676, -223.5124) -> (88.8809, -218.5124)
  line L581 (87.4375, -181.0124) -> (84.5507, -186.0124)
  line L582 (78.7772, -186.0124) -> (75.8905, -181.0124)
  line L583 (84.5507, -186.0124) -> (78.7772, -186.0124)
  line L584 (84.5507, -191.0124) -> (87.4375, -196.0124)
  line L585 (75.8905, -196.0124) -> (78.7772, -191.0124)
  line L586 (87.4375, -196.0124) -> (84.5507, -201.0124)
  line L587 (78.7772, -201.0124) -> (75.8905, -196.0124)
  line L588 (84.5507, -201.0124) -> (78.7772, -201.0124)
  line L589 (78.7772, -191.0124) -> (84.5507, -191.0124)
  line L590 (100.4279, -203.5124) -> (97.5411, -208.5124)
  line L591 (97.5411, -198.5124) -> (100.4279, -203.5124)
  line L592 (110.5507, -176.0124) -> (113.4375, -181.0124)
  line L593 (104.7772, -176.0124) -> (110.5507, -176.0124)
  line L594 (101.8905, -181.0124) -> (104.7772, -176.0124)
  line L595 (123.5411, -208.5124) -> (117.7676, -208.5124)
  line L596 (117.7676, -198.5124) -> (123.5411, -198.5124)
  line L597 (126.4279, -188.5124) -> (123.5411, -193.5124)
  line L598 (123.5411, -193.5124) -> (117.7676, -193.5124)
  line L599 (123.5411, -183.5124) -> (126.4279, -188.5124)
  line L600 (117.7676, -183.5124) -> (123.5411, -183.5124)
  line L601 (117.7676, -208.5124) -> (114.8809, -203.5124)
  line L602 (114.8809, -203.5124) -> (117.7676, -198.5124)
  line L603 (117.7676, -193.5124) -> (114.8809, -188.5124)
  line L604 (114.8809, -188.5124) -> (117.7676, -183.5124)
  line L605 (113.4375, -211.0124) -> (110.5507, -216.0124)
  line L606 (110.5507, -221.0124) -> (113.4375, -226.0124)
  line L607 (113.4375, -226.0124) -> (110.5507, -231.0124)
  line L608 (104.7772, -221.0124) -> (110.5507, -221.0124)
  line L609 (110.5507, -231.0124) -> (104.7772, -231.0124)
  line L610 (104.7772, -231.0124) -> (101.8905, -226.0124)
  line L611 (101.8905, -226.0124) -> (104.7772, -221.0124)
  line L612 (110.5507, -206.0124) -> (113.4375, -211.0124)
  line L613 (110.5507, -216.0124) -> (104.7772, -216.0124)
  line L614 (104.7772, -216.0124) -> (101.8905, -211.0124)
  line L615 (104.7772, -206.0124) -> (110.5507, -206.0124)
  line L616 (101.8905, -211.0124) -> (104.7772, -206.0124)
  line L617 (114.8809, -218.5124) -> (117.7676, -213.5124)
  line L618 (117.7676, -213.5124) -> (123.5411, -213.5124)
  line L619 (123.5411, -213.5124) -> (126.4279, -218.5124)
  line L620 (123.5411, -223.5124) -> (117.7676, -223.5124)
  line L621 (126.4279, -218.5124) -> (123.5411, -223.5124)
  line L622 (117.7676, -223.5124) -> (114.8809, -218.5124)
  line L623 (113.4375, -181.0124) -> (110.5507, -186.0124)
  line L624 (104.7772, -186.0124) -> (101.8905, -181.0124)
  line L625 (110.5507, -186.0124) -> (104.7772, -186.0124)
  line L626 (110.5507, -191.0124) -> (113.4375, -196.0124)
  line L627 (101.8905, -196.0124) -> (104.7772, -191.0124)
  line L628 (113.4375, -196.0124) -> (110.5507, -201.0124)
  line L629 (104.7772, -201.0124) -> (101.8905, -196.0124)
  line L630 (110.5507, -201.0124) -> (104.7772, -201.0124)
  line L631 (104.7772, -191.0124) -> (110.5507, -191.0124)
  line L632 (126.4279, -203.5124) -> (123.5411, -208.5124)
  line L633 (123.5411, -198.5124) -> (126.4279, -203.5124)
  line L634 (136.5507, -176.0124) -> (139.4375, -181.0124)
  line L635 (130.7772, -176.0124) -> (136.5507, -176.0124)
  line L636 (127.8905, -181.0124) -> (130.7772, -176.0124)
  line L637 (149.5411, -208.5124) -> (143.7676, -208.5124)
  line L638 (143.7676, -198.5124) -> (149.5411, -198.5124)
  line L639 (152.4279, -188.5124) -> (149.5411, -193.5124)
  line L640 (149.5411, -193.5124) -> (143.7676, -193.5124)
  line L641 (149.5411, -183.5124) -> (152.4279, -188.5124)
  line L642 (143.7676, -183.5124) -> (149.5411, -183.5124)
  line L643 (143.7676, -208.5124) -> (140.8809, -203.5124)
  line L644 (140.8809, -203.5124) -> (143.7676, -198.5124)
  line L645 (143.7676, -193.5124) -> (140.8809, -188.5124)
  line L646 (140.8809, -188.5124) -> (143.7676, -183.5124)
  line L647 (139.4375, -211.0124) -> (136.5507, -216.0124)
  line L648 (136.5507, -221.0124) -> (139.4375, -226.0124)
  line L649 (139.4375, -226.0124) -> (136.5507, -231.0124)
  line L650 (130.7772, -221.0124) -> (136.5507, -221.0124)
  line L651 (136.5507, -231.0124) -> (130.7772, -231.0124)
  line L652 (130.7772, -231.0124) -> (127.8905, -226.0124)
  line L653 (127.8905, -226.0124) -> (130.7772, -221.0124)
  line L654 (136.5507, -206.0124) -> (139.4375, -211.0124)
  line L655 (136.5507, -216.0124) -> (130.7772, -216.0124)
  line L656 (130.7772, -216.0124) -> (127.8905, -211.0124)
  line L657 (130.7772, -206.0124) -> (136.5507, -206.0124)
  line L658 (127.8905, -211.0124) -> (130.7772, -206.0124)
  line L659 (140.8809, -218.5124) -> (143.7676, -213.5124)
  line L660 (143.7676, -213.5124) -> (149.5411, -213.5124)
  line L661 (149.5411, -213.5124) -> (152.4279, -218.5124)
  line L662 (149.5411, -223.5124) -> (143.7676, -223.5124)
  line L663 (152.4279, -218.5124) -> (149.5411, -223.5124)
  line L664 (143.7676, -223.5124) -> (140.8809, -218.5124)
  line L665 (139.4375, -181.0124) -> (136.5507, -186.0124)
  line L666 (130.7772, -186.0124) -> (127.8905, -181.0124)
  line L667 (136.5507, -186.0124) -> (130.7772, -186.0124)
  line L668 (136.5507, -191.0124) -> (139.4375, -196.0124)
  line L669 (127.8905, -196.0124) -> (130.7772, -191.0124)
  line L670 (139.4375, -196.0124) -> (136.5507, -201.0124)
  line L671 (130.7772, -201.0124) -> (127.8905, -196.0124)
  line L672 (136.5507, -201.0124) -> (130.7772, -201.0124)
  line L673 (130.7772, -191.0124) -> (136.5507, -191.0124)
  line L674 (152.4279, -203.5124) -> (149.5411, -208.5124)
  line L675 (149.5411, -198.5124) -> (152.4279, -203.5124)
  line L676 (162.5507, -176.0124) -> (165.4375, -181.0124)
  line L677 (156.7772, -176.0124) -> (162.5507, -176.0124)
  line L678 (153.8905, -181.0124) -> (156.7772, -176.0124)
  line L679 (175.5411, -208.5124) -> (169.7676, -208.5124)
  line L680 (169.7676, -198.5124) -> (175.5411, -198.5124)
  line L681 (178.4279, -188.5124) -> (175.5411, -193.5124)
  line L682 (175.5411, -193.5124) -> (169.7676, -193.5124)
  line L683 (175.5411, -183.5124) -> (178.4279, -188.5124)
  line L684 (169.7676, -183.5124) -> (175.5411, -183.5124)
  line L685 (169.7676, -208.5124) -> (166.8809, -203.5124)
  line L686 (166.8809, -203.5124) -> (169.7676, -198.5124)
  line L687 (169.7676, -193.5124) -> (166.8809, -188.5124)
  line L688 (166.8809, -188.5124) -> (169.7676, -183.5124)
  line L689 (165.4375, -211.0124) -> (162.5507, -216.0124)
  line L690 (162.5507, -221.0124) -> (165.4375, -226.0124)
  line L691 (165.4375, -226.0124) -> (162.5507, -231.0124)
  line L692 (156.7772, -221.0124) -> (162.5507, -221.0124)
  line L693 (162.5507, -231.0124) -> (156.7772, -231.0124)
  line L694 (156.7772, -231.0124) -> (153.8905, -226.0124)
  line L695 (153.8905, -226.0124) -> (156.7772, -221.0124)
  line L696 (162.5507, -206.0124) -> (165.4375, -211.0124)
  line L697 (162.5507, -216.0124) -> (156.7772, -216.0124)
  line L698 (156.7772, -216.0124) -> (153.8905, -211.0124)
  line L699 (156.7772, -206.0124) -> (162.5507, -206.0124)
  line L700 (153.8905, -211.0124) -> (156.7772, -206.0124)
  line L701 (166.8809, -218.5124) -> (169.7676, -213.5124)
  line L702 (169.7676, -213.5124) -> (175.5411, -213.5124)
  line L703 (175.5411, -213.5124) -> (178.4279, -218.5124)
  line L704 (175.5411, -223.5124) -> (169.7676, -223.5124)
  line L705 (178.4279, -218.5124) -> (175.5411, -223.5124)
  line L706 (169.7676, -223.5124) -> (166.8809, -218.5124)
  line L707 (165.4375, -181.0124) -> (162.5507, -186.0124)
  line L708 (156.7772, -186.0124) -> (153.8905, -181.0124)
  line L709 (162.5507, -186.0124) -> (156.7772, -186.0124)
  line L710 (162.5507, -191.0124) -> (165.4375, -196.0124)
  line L711 (153.8905, -196.0124) -> (156.7772, -191.0124)
  line L712 (165.4375, -196.0124) -> (162.5507, -201.0124)
  line L713 (156.7772, -201.0124) -> (153.8905, -196.0124)
  line L714 (162.5507, -201.0124) -> (156.7772, -201.0124)
  line L715 (156.7772, -191.0124) -> (162.5507, -191.0124)
  line L716 (178.4279, -203.5124) -> (175.5411, -208.5124)
  line L717 (175.5411, -198.5124) -> (178.4279, -203.5124)
  line L718 (188.5507, -176.0124) -> (191.4375, -181.0124)
  line L719 (182.7772, -176.0124) -> (188.5507, -176.0124)
  line L720 (179.8905, -181.0124) -> (182.7772, -176.0124)
  line L721 (201.5411, -208.5124) -> (195.7676, -208.5124)
  line L722 (195.7676, -198.5124) -> (201.5411, -198.5124)
  line L723 (204.4279, -188.5124) -> (201.5411, -193.5124)
  line L724 (201.5411, -193.5124) -> (195.7676, -193.5124)
  line L725 (201.5411, -183.5124) -> (204.4279, -188.5124)
  line L726 (195.7676, -183.5124) -> (201.5411, -183.5124)
  line L727 (195.7676, -208.5124) -> (192.8809, -203.5124)
  line L728 (192.8809, -203.5124) -> (195.7676, -198.5124)
  line L729 (195.7676, -193.5124) -> (192.8809, -188.5124)
  line L730 (192.8809, -188.5124) -> (195.7676, -183.5124)
  line L731 (191.4375, -211.0124) -> (188.5507, -216.0124)
  line L732 (188.5507, -221.0124) -> (191.4375, -226.0124)
  line L733 (191.4375, -226.0124) -> (188.5507, -231.0124)
  line L734 (182.7772, -221.0124) -> (188.5507, -221.0124)
  line L735 (188.5507, -231.0124) -> (182.7772, -231.0124)
  line L736 (182.7772, -231.0124) -> (179.8905, -226.0124)
  line L737 (179.8905, -226.0124) -> (182.7772, -221.0124)
  line L738 (188.5507, -206.0124) -> (191.4375, -211.0124)
  line L739 (188.5507, -216.0124) -> (182.7772, -216.0124)
  line L740 (182.7772, -216.0124) -> (179.8905, -211.0124)
  line L741 (182.7772, -206.0124) -> (188.5507, -206.0124)
  line L742 (179.8905, -211.0124) -> (182.7772, -206.0124)
  line L743 (192.8809, -218.5124) -> (195.7676, -213.5124)
  line L744 (195.7676, -213.5124) -> (201.5411, -213.5124)
  line L745 (201.5411, -213.5124) -> (204.4279, -218.5124)
  line L746 (201.5411, -223.5124) -> (195.7676, -223.5124)
  line L747 (204.4279, -218.5124) -> (201.5411, -223.5124)
  line L748 (195.7676, -223.5124) -> (192.8809, -218.5124)
  line L749 (191.4375, -181.0124) -> (188.5507, -186.0124)
  line L750 (182.7772, -186.0124) -> (179.8905, -181.0124)
  line L751 (188.5507, -186.0124) -> (182.7772, -186.0124)
  line L752 (188.5507, -191.0124) -> (191.4375, -196.0124)
  line L753 (179.8905, -196.0124) -> (182.7772, -191.0124)
  line L754 (191.4375, -196.0124) -> (188.5507, -201.0124)
  line L755 (182.7772, -201.0124) -> (179.8905, -196.0124)
  line L756 (188.5507, -201.0124) -> (182.7772, -201.0124)
  line L757 (182.7772, -191.0124) -> (188.5507, -191.0124)
  line L758 (204.4279, -203.5124) -> (201.5411, -208.5124)
  line L759 (201.5411, -198.5124) -> (204.4279, -203.5124)
  line L760 (214.5507, -176.0124) -> (217.4375, -181.0124)
  line L761 (208.7772, -176.0124) -> (214.5507, -176.0124)
  line L762 (205.8905, -181.0124) -> (208.7772, -176.0124)
  line L763 (227.5411, -208.5124) -> (221.7676, -208.5124)
  line L764 (221.7676, -198.5124) -> (227.5411, -198.5124)
  line L765 (230.4279, -188.5124) -> (227.5411, -193.5124)
  line L766 (227.5411, -193.5124) -> (221.7676, -193.5124)